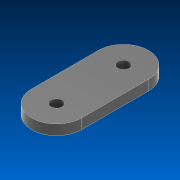
# Autodesk Inventor part: Small Motor Spacer
Saved by Autodesk Inventor 2022.2 (Build 262287000, 287)
## iProperties
Created: 2022-01-05
Part Number: Small Motor Spacer
Material: PET Plastic
Document SubType Name: Modeling
Designer: omard
Density: 1.541 g/cm^3
Appearance: Smooth - Black
Author: omard
Autodesk Inventor part; units mm, degrees
ref_plane "YZ Plane" through (0, 0, 0) normal (1, 0, 0) x (0, 1, 0)
ref_plane "XZ Plane" through (0, 0, 0) normal (0, 1, 0) x (-1, 0, 0)
ref_plane "XY Plane" through (0, 0, 0) normal (0, 0, 1) x (1, 0, 0)
sketch "Sketch1" plane through (0, 0, 0) normal (0, 1, 0) x (-1, 0, 0)
  circle A0 centre (0, 0) radius 2.159
  circle A1 centre (0, -25.4) radius 2.159
  line L0 (0, 0) -> (0, -25.4) construction
  line L1 (-9.525, 0) -> (-9.525, -25.4)
  line L2 (9.525, -25.4) -> (9.525, 0)
  arc A2 (9.525, 0) -> (-9.525, 0) centre (0, 0) ccw
  arc A3 (-9.525, -25.4) -> (9.525, -25.4) centre (0, -25.4) ccw
  point P0 (0, -12.7)
  dimension "d0" = 4.318
  dimension "d2" = 25.4
  dimension "d3" = 19.05
  constraints: 8 end point, 4 centre point, 4 point on circle, 4 tangent, 1 coincident, 1 equal radius, 1 midpoint, 1 parallel, 1 vertical, 1 vertical alignment
  measures "d0" diameter of A0
  measures "d2" distance of L0.end point (0, 0)
  measures "d3" diameter of A3
extrude "Extrusion1" add sketch "Sketch1" along normal blind 3.861
body "Solid1"
